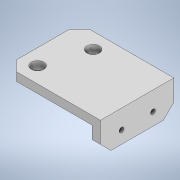
# Autodesk Inventor part: Peça29
Saved by Autodesk Inventor 2021 (Build 250183000, 183)
## iProperties
Created: 2021-07-21
Part Number: Peça29
Material: Genérico
Document SubType Name: Modeling
Designer: Giovanni
Density: 1 g/cm^3
Appearance: Padrão
Author: Giovanni
Autodesk Inventor part; units mm, degrees
ref_plane "YZ Plane" through (0, 0, 0) normal (1, 0, 0) x (0, 1, 0)
ref_plane "XZ Plane" through (0, 0, 0) normal (0, 1, 0) x (-1, 0, 0)
ref_plane "XY Plane" through (0, 0, 0) normal (0, 0, 1) x (1, 0, 0)
sketch "Esboço1" plane through (0, 0, 0) normal (0, 0, 1) x (1, 0, 0)
  line L0 (-90, 0) -> (0, 0)
  line L1 (0, 0) -> (0, -30)
  line L2 (0, -30) -> (-8, -30)
  line L3 (-8, -30) -> (-8, -8)
  line L4 (-8, -8) -> (-90, -8)
  line L5 (-90, -8) -> (-90, 0)
  dimension "d0" = 90
  dimension "d1" = 30
  dimension "d2" = 8
  dimension "d3" = 8
  constraints: 12 end point, 4 perpendicular, 1 horizontal, 1 vertical
  measures "d0" distance of L0.start L0.end
  measures "d1" distance of L0.end L1.end
  measures "d2" distance of L1.end L2.end
  measures "d3" distance of L4.end L0.start
extrude "Extrusão1" add sketch "Esboço1" along normal mid plane 70
sketch "Esboço2" plane through (-90, 0, 35) normal (0, 1, 0) x (1, 0, 0)
  line L0 (0, 70) -> (0, 0) projected
  line L1 (90, 0) -> (0, 0) projected
  line L2 (0, 70) -> (90, 70) projected
  point P0 (90, 35)
  point P1 (28, 55)
  point P2 (15, 15)
  dimension "d6" = 28
  dimension "d7" = 15
  dimension "d8" = 15
  dimension "d9" = 15
  measures "d6" horizontal distance of L0.end point (28, 55)
  measures "d7" distance from line of L0 point (15, 15)
  measures "d8" distance from line of point (15, 15) L1
  measures "d9" distance from line of L2 point (28, 55)
hole "Furo1" at (-62, 0, -20) at (-75, 0, 20) direction (0, -1, 0) diameter 12 end through all
sketch "Esboço3" plane through (-8, -30, 35) normal (-1, 0, 0) x (0, 0, 1)
  line L0 (-70, 0) -> (0, 0) projected
  line L1 (0, 22) -> (0, 0) projected
  line L2 (-70, 0) -> (-70, 22) projected
  point P0 (-35, 30)
  point P1 (-50, 12)
  point P2 (-20, 12)
  dimension "d17" = 12
  dimension "d18" = 20
  dimension "d19" = 20
  constraints: 1 horizontal alignment
  measures "d17" distance from line of L0 point (-50, 12)
  measures "d18" distance from line of point (-20, 12) L1
  measures "d19" distance from line of L2 point (-50, 12)
hole "Furo2" at (-8, -18, -15) at (-8, -18, 15) direction (1, 0, 0) diameter 4.5 end through all
chamfer "Chanfro1" distance 10 angle 45 4 edges at (-90, -4, -35) (-90, -4, 35) (-4, -30, -35) (-4, -30, 35)
